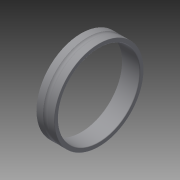
# Autodesk Inventor part: A-2418_ir
Saved by Autodesk Inventor 2014 SP2 (Build 180246200, 246)
## iProperties
Created: 2019-11-12
Part Number: A-2418_ir
Material: Generic
Catalog Web Link: www.cadenas.de
Description: Radial Ball Bearings (A series)  OT ir-Radial Ball Bearings (A series)  Open Type
Vendor: NMB
Document SubType Name: Modeling
Designer: psadmin
Manufacturer: NMB
Mass: 0.199901 g
Surface Area: 5.70856 cm^2
Volume: 0.199901 cm^3
Density: 1 g/cm^3
Appearance: PSOLRGB-192-192-192
Category: PARTsolutions
Company: NMB
Title: A-2418_ir
Author: Cadenas PARTsolutions
Comments: Radial Ball Bearings (A series)  Open Type
PSOL_IDENT_0: {$CADENAS_DATA\23d-libs\nmb\pbbp\radial_ball_bear_thin_secti\rbb_as\as_open_ir.prj},191 {VTYP=3D},{N
PSOL_IDENT_1: B=A-2418_ir},{LINA=A-2418_ir},{NN=Radial Ball Bearings (A series)  OT ir},{DATE=11.11.2013 05:13:38}
PSOL_IDENT_2: ,{GEOMDATE=29.10.2013 14:08:00},{VERSION=},{LINEID=890},{WBVAR=},{WBNUMERIC=}  {NB=A-2418_ir},{LINA=
PSOL_IDENT_3: A-2418_ir},{KT=DUMMY},{IDNR=},{PN=A-2418},{SHLD=open},{FLANG=unflanged},{SD=18.000},{D=24.000},{B=4.
PSOL_IDENT_4: 000},{SR=0.15},{BCZ=16},{DW=1.5875},{LI=19.75},{LO=21.93},{D1=0.000},{C1=0.00},{D2=0.0},{C2=0.00},{C
PSOL_IDENT_5: OR=654},{CR=1087},{PCD=21.000},{U=22.588},{W=19.413},{Y=0.794},{Z=0.794},{AA=0.000},{AC=0.00},{AD=0.
PSOL_IDENT_6: 000},{AF=0.00},{AQ=0.00},{AH=0.00},{AI=0.00},{AJ=0.00}
NN: Radial Ball Bearings (A series)  OT ir
NT: Radial Ball Bearings (A series)  Open Type
NB: A-2418_ir
NBSYN: $PN._ir
LINA: A-2418_ir
PN: A-2418
SHLD: open
FLANG: unflanged
SD: 18
D: 24
B: 4
SR: 0.15
BCZ: 16
DW: 1.5875
LI: 19.75
LO: 21.93
D1: 0
C1: 0
D2: 0
C2: 0
COR: 654
CR: 1087
PCD: 21
U: 22.588
W: 19.413
Y: 0.794
Z: 0.794
AA: 0
AC: 0
AD: 0
AF: 0
AQ: 0
AH: 0
AI: 0
AJ: 0
SUPPLIER: NMB
ARTICLENO: A-2418_ir
BOMINFO: A-2418_ir
CREATOR: CADENAS GmbH
Autodesk Inventor part; units mm, degrees
sketch "Sketch_1" plane through (0, 0, 0) normal (0, 0, 1) x (1, 0, 0)
  line L0 (4, 0) -> (0, 0)
  line L1 (0, 9.8) -> (0, 9.15)
  arc A0 (0, 9.15) -> (0.15, 9) centre (0.15, 9.15) ccw
  line L2 (0.15, 9) -> (3.85, 9)
  arc A1 (3.85, 9) -> (4, 9.15) centre (3.85, 9.15) ccw
  line L3 (4, 9.15) -> (4, 9.8)
  arc A2 (4, 9.8) -> (3.925, 9.875) centre (3.925, 9.8) ccw
  line L4 (3.925, 9.875) -> (2.4893, 9.875)
  arc A3 (1.5107, 9.875) -> (2.4893, 9.875) centre (2, 10.5) ccw
  line L5 (1.5107, 9.875) -> (0.075, 9.875)
  arc A4 (0.075, 9.875) -> (0, 9.8) centre (0.075, 9.8) ccw
  constraints: 12 end point, 10 point on circle, 5 centre point
revolve "Revolution1" add sketch "Sketch_1" angle 360 about axis through (4, 0, 0) along (1, 0, 0)
ref_plane "1_XY" through (2, 0, 0) normal (1, 0, 0) x (0, 0, -1)
ref_plane "1_YZ" through (2, 0, 0) normal (0, 0, -1) x (0, 1, 0)
ref_plane "1_ZX" through (2, 0, 0) normal (0, 1, 0) x (1, 0, 0)
ref_plane "1_Dummy_XY" through (0, 0, 0) normal (-1, 0, 0) x (0, 0, -1)
ref_plane "1_Dummy_YZ" through (0, 0, 0) normal (0, 0, -1) x (0, -1, 0)
ref_plane "1_Dummy_ZX" through (0, 0, 0) normal (0, -1, 0) x (-1, 0, 0)
body "Solid1"
